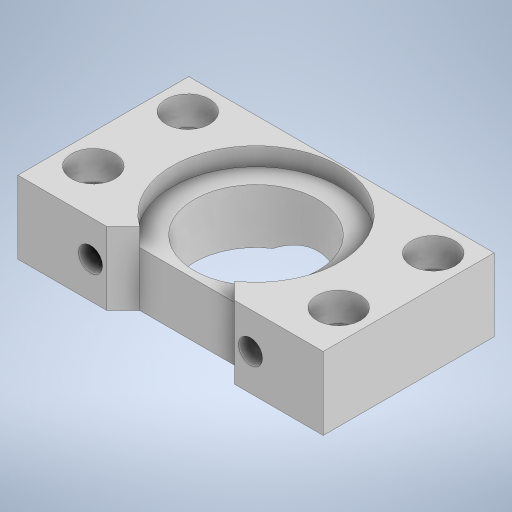
# Autodesk Inventor part: y_motor_lock_top2
Saved by Autodesk Inventor 2023 (Build 270158030, 158C)
## iProperties
Created: 2022-05-11
Part Number: y_motor_lock_top2
Material: 一般
Document SubType Name: Modeling
Designer: user
Density: 1 g/cm^3
Appearance: 預設
Author: user
## iProperties of the stored document y_motor_lock_top2_3D 列印.ipt
Created: 2022-05-15
Part Number: y_motor_lock_top2_3D 列印
Material: 一般
Document SubType Name: Modeling
Designer: user
Density: 1 g/cm^3
Appearance: 預設
Author: user
Autodesk Inventor part; units mm, degrees
ref_plane "YZ Plane" through (0, 0, 0) normal (1, 0, 0) x (0, 1, 0)
ref_plane "XZ Plane" through (0, 0, 0) normal (0, 1, 0) x (-1, 0, 0)
ref_plane "XY Plane" through (0, 0, 0) normal (0, 0, 1) x (1, 0, 0)
sketch "草圖4" plane through (0, 0, 0) normal (0, 0, 1) x (1, 0, 0)
  line L0 (-29.4, 0) -> (29.4, 0) projected
  line L1 (0, -7) -> (0, 7) projected
  line L2 (-21, 5) -> (21, 5)
  line L3 (21, 5) -> (21, -5)
  line L4 (21, -5) -> (-21, -5)
  line L5 (-21, -5) -> (-21, 5)
  circle A0 centre (-11, 0) radius 1.65
  circle A1 centre (11, 0) radius 1.65
  point P0 (0, 0)
  dimension "d20" = 42
  dimension "d21" = 10
  dimension "d22" = 3.3
  dimension "d23" = 3.3
  dimension "d24" = 10
  dimension "d25" = 10
  constraints: 8 end point, 2 centre point, 2 parallel, 2 point on line, 1 horizontal, 1 perpendicular, 2 other
  measures "d20" distance of L3.end L4.end
  measures "d21" distance of L2.end L3.end
  measures "d22" diameter of A0
  measures "d23" diameter of A1
  measures "d24" distance from line of L5 A0.centre
  measures "d25" distance from line of L3 A1.centre
extrude "擠出3" add sketch "草圖4" along normal mid plane 23.5 contours L5 L2 L1 L0 A0 | L0 A0 L1 L4 L5 | L1 L0 A1 L3 L4 | L2 L3 L0 A1 L1
sketch "草圖5" plane through (-21, 5, 11.75) normal (0, 1, 0) x (1, 0, 0)
  line L0 (0, 0) -> (0, 23.5) projected
  line L1 (42, 0) -> (0, 0) projected
  line L2 (42, 23.5) -> (42, 0) projected
  line L3 (0, 23.5) -> (42, 23.5) projected
  circle A0 centre (21, 11.75) radius 8.5
  circle A1 centre (4.125, 19.25) radius 1.65
  circle A2 centre (4.125, 6.25) radius 1.65
  line L4 (42, 23.5) -> (0, 23.5) projected
  line L5 (21, 23.5) -> (21, 25.0136)
  circle A3 centre (37.875, 19.25) radius 1.65
  circle A4 centre (37.875, 6.25) radius 1.65
  circle A5 centre (4.125, 19.25) radius 3
  circle A6 centre (4.125, 6.25) radius 3
  circle A7 centre (37.875, 19.25) radius 3
  circle A8 centre (37.875, 6.25) radius 3
  dimension "d28" = 17
  dimension "d31" = 3.3
  dimension "d32" = 3.3
  dimension "d33" = 4.125
  dimension "d34" = 4.25
  dimension "d35" = 6.25
  dimension "d36" = 4.125
  dimension "d37" = 6
  dimension "d38" = 6
  constraints: 9 centre point, 4 symmetric about line, 3 coincident, 2 end point, 1 midpoint, 1 vertical, 4 other
  measures "d28" diameter of A0
  measures "d31" diameter of A1
  measures "d32" diameter of A2
  measures "d33" distance from line of L0 A1.centre
  measures "d34" distance from line of L3 A1.centre
  measures "d35" distance from line of L1 A2.centre
  measures "d36" distance from line of L0 A2.centre
  measures "d37" diameter of A5
  measures "d38" diameter of A6
extrude "擠出4" cut sketch "草圖5" against normal up to surface (10 mm away) contours A0 | A1 | A2 | A3 | A4
extrude "擠出5" cut sketch "草圖5" against normal blind 4 contours A5 | A6 | A7 | A8
sketch "草圖7" plane through (0, 0, -11.75) normal (0, 0, -1) x (-1, 0, 0)
  circle A0 centre (11, 0) radius 2.75 projected
  circle A1 centre (-11, 0) radius 2.75 projected
  arc A2 (5, -4) -> (-5, -4) centre (0, -12.6603) ccw projected
  line L0 (18.5, -4) -> (5, -4) projected
  line L1 (18.5, -4) -> (18.5, 4) projected
  line L2 (18.5, 4) -> (-18.5, 4) projected
  line L3 (-18.5, 4) -> (-18.5, -4) projected
  line L4 (-5, -4) -> (-18.5, -4) projected
  line L5 (21, -5) -> (21, 5) projected
  line L6 (21, 5) -> (-21, 5) projected
  line L7 (-21, 5) -> (-21, -5) projected
  line L8 (-21, -5) -> (21, -5) projected
  circle A3 centre (-11, 0) radius 1.65 projected
  circle A4 centre (11, 0) radius 1.65 projected
  arc A5 (4.7245, -5) -> (-4.7245, -5) centre (0, -12.6603) ccw
  line L9 (4.7245, -5) -> (19.5, -5)
  line L10 (19.5, -5) -> (19.5, 5)
  line L11 (19.5, 5) -> (-19.5, 5)
  line L12 (-19.5, 5) -> (-19.5, -5)
  line L13 (-19.5, -5) -> (-4.7245, -5)
  point P0 (0, 0)
  point P1 (-5, -4)
  point P2 (5, -4)
  point P3 (-4.7245, -5)
  constraints: 10 end point, 2 point on circle, 1 centre point, 1 point on line, 5 other
extrude "擠出7" cut sketch "草圖7" against normal blind 8.65 contours L8 A5
sketch "草圖8" plane through (-21, 5, 11.75) normal (0, 1, 0) x (1, 0, 0)
  circle A0 centre (37.875, 6.25) radius 3 projected
  circle A1 centre (4.125, 6.25) radius 3 projected
  circle A2 centre (21, 11.75) radius 8.5 projected
  line L0 (0, 0) -> (0, 23.5) projected
  line L1 (42, 0) -> (0, 0) projected
  line L2 (42, 23.5) -> (42, 0) projected
  circle A3 centre (21, 11.75) radius 11.5
  line L3 (0, 23.5) -> (42, 23.5) projected
  dimension "d45" = 23
  constraints: 1 centre point, 1 coincident
  measures "d45" diameter of A3
extrude "擠出8" cut sketch "草圖8" against normal blind 2.5 contours A0 | A1 | A2 | A3
sketch "草圖10" plane through (-21, 5, 11.75) normal (0, 1, 0) x (1, 0, 0)
  circle A0 centre (26.5805, -1.1666) radius 1.5 projected
  circle A1 centre (26.5805, -1.1666) radius 2.75
  point P0 (21, 11.75)
  dimension "d55" = 5.5
  constraints: 1 centre point, 1 coincident
  measures "d55" diameter of A1
extrude "擠出10" cut sketch "草圖10" against normal up to surface (10 mm away) contours A0 | A1
sketch "草圖11" plane through (-21, 5, -11.75) normal (0, 1, 0) x (1, 0, 0)
  circle A0 centre (15.3833, -24.75) radius 1.5
  circle A1 centre (15.3833, -24.75) radius 2.75
  point P0 (21, -11.75)
  dimension "d58" = 5.5
  constraints: 2 centre point, 1 coincident, 2 other
  measures "d58" diameter of A1
extrude "擠出11" cut sketch "草圖11" against normal up to surface (10 mm away) contours A0 | A1
sketch "草圖12" plane through (-21, 5, -11.75) normal (0, 1, 0) x (1, 0, 0)
  arc A0 (15.8732, -22.044) -> (12.9338, -23.5) centre (15.3833, -24.75) ccw projected
  arc A1 (26.3579, -21.9256) -> (15.8732, -22.044) centre (21, -11.75) ccw projected
  arc A2 (29.0708, -23.5) -> (26.3579, -21.9256) centre (26.5805, -24.6666) ccw projected
  line L0 (42, -23.5) -> (29.0708, -23.5) projected
  line L1 (42, 0) -> (42, -23.5) projected
  line L2 (0, 0) -> (42, 0) projected
  line L3 (0, -23.5) -> (0, 0) projected
  line L4 (12.9338, -23.5) -> (0, -23.5) projected
  circle A3 centre (37.875, -17.25) radius 3 projected
  circle A4 centre (4.125, -17.25) radius 3 projected
  circle A5 centre (37.875, -4.25) radius 3 projected
  circle A6 centre (4.125, -4.25) radius 3 projected
  line L5 (42, -23.5) -> (29.0708, -23.5) projected
  line L6 (29.7708, -23.5) -> (12.2338, -23.5)
  line L7 (12.2338, -23.5) -> (12.2338, -21.2337)
  line L8 (12.2338, -21.2337) -> (29.7708, -21.2337)
  line L9 (29.7708, -21.2337) -> (29.7708, -23.5)
  line L10 (29.7708, -23.5) -> (27.5045, -21.2337)
  line L11 (29.7708, -23.5) -> (32.9758, -23.5) construction
  line L12 (12.2338, -23.5) -> (14.5001, -21.2337)
  line L13 (12.2338, -23.5) -> (15.4388, -23.5) construction
  arc A7 (26.3579, -21.9256) -> (15.8732, -22.044) centre (21, -11.75) ccw projected
  point P0 (12.9338, -23.5)
  dimension "d62" = 0.7
  dimension "d63" = 0.7
  dimension "d64" = 135
  dimension "d65" = 45
  constraints: 16 end point, 3 horizontal, 3 point on line, 2 equal length, 2 parallel, 1 perpendicular, 1 point on circle
  measures "d62" distance from line of L9 L0.end
  measures "d63" distance from line of L4.start L7
  measures "d64" angle of L11 L10
  measures "d65" angle of L13 L12
extrude "擠出12" cut sketch "草圖12" against normal up to surface (10 mm away) contours A1 L8 A2 L6 A0 | A0 L4 L12 A1 | A2 A1 L10 L0
